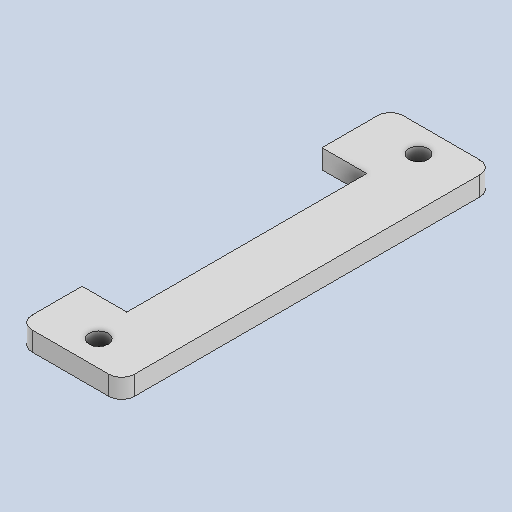
# Autodesk Inventor part: projectorPlace
Saved by Autodesk Inventor 2024 (Build 280153000, 153)
## iProperties
Created: 2021-07-13
Part Number: projectorPlace
Material: Generic
Document SubType Name: Modeling
Designer: dsdan
Density: 1 g/cm^3
Appearance: Default
Author: dsdan
Autodesk Inventor part; units mm, degrees
ref_plane "YZ Plane" through (0, 0, 0) normal (1, 0, 0) x (0, 1, 0)
ref_plane "XZ Plane" through (0, 0, 0) normal (0, 1, 0) x (-1, 0, 0)
ref_plane "XY Plane" through (0, 0, 0) normal (0, 0, 1) x (1, 0, 0)
sketch "Sketch1" plane through (0, 0, 0) normal (0, 1, 0) x (-1, 0, 0)
  line L0 (-7.9182, -1.6904) -> (24.0818, -1.6904)
  line L1 (24.0818, -1.6904) -> (24.0818, -21.3281)
  line L2 (24.0818, -21.3281) -> (10.0818, -21.3281)
  line L3 (-7.9182, -21.3281) -> (-7.9182, -1.6904)
  line L4 (10.0818, -21.3281) -> (10.0818, -96.3281)
  line L5 (-7.9182, -96.3281) -> (-7.9182, -21.3281)
  line L6 (10.0818, -96.3281) -> (24.0818, -96.3281)
  line L7 (24.0818, -96.3281) -> (24.0818, -117.6904)
  line L8 (24.0818, -117.6904) -> (-7.9182, -117.6904)
  line L9 (-7.9182, -117.6904) -> (-7.9182, -96.3281)
  circle A0 centre (7.2678, -9.6904) radius 3
  circle A1 centre (7.2678, -109.6904) radius 3
  circle A2 centre (7.2678, -9.6904) radius 2.5 projected
  circle A3 centre (7.2678, -109.6904) radius 2.5 projected
  line L10 (60.0818, -21.3281) -> (10.0818, -21.3281) projected
  line L11 (60.0818, -96.3281) -> (10.0818, -96.3281) projected
  line L12 (10.0818, -71.5281) -> (10.0818, -46.1281) projected
  point P0 (13.365, -96.3281)
  point P1 (13.365, -21.3281)
  point P2 (-7.9182, -57.2241)
  point P3 (-7.9182, -21.3281)
  point P4 (-7.9182, -21.3281)
  point P5 (-7.9182, -96.3281)
  point P6 (-7.9182, -96.3281)
  dimension "d3" = 6
  dimension "d4" = 6
  dimension "d5" = 32
  dimension "d12" = 18
  dimension "d13" = 8
  dimension "d14" = 8
  constraints: 20 end point, 5 parallel, 3 collinear, 2 centre point, 2 concentric, 2 horizontal, 2 perpendicular, 1 point on line
  measures "d3" diameter of A0
  measures "d4" diameter of A1
  measures "d5" distance of L0.start L0.end
  measures "d12" distance between parallel lines of L4 L5
  measures "d13" distance from line of A0.centre L0
  measures "d14" distance from line of A1.centre L8
extrude "Extrusion1" add sketch "Sketch1" along normal blind 6 contours L0 L1 L2 L4 L6 L7 L8 L9 L5 L3
fillet "Fillet1" radius 4 4 edges at (7.9182, 3, -1.6904) (7.9182, 3, -117.6904) (-24.0818, 3, -117.6904) (-24.0818, 3, -1.6904)
equation "\"d14\" = d13"
equation "\"d1\" = d3"
body "Solid1"
